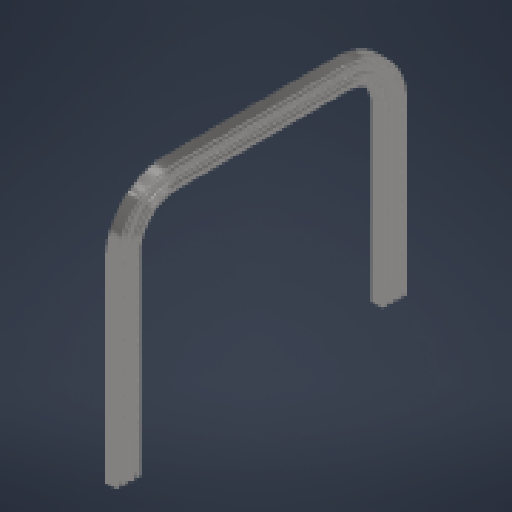
# Autodesk Inventor part: SACMI DPA C-RAIL
Saved by Autodesk Inventor 2025 (Build 290162000, 162)
## iProperties
Created: 2024-05-16
Part Number: SACMI DPA C-RAIL
Material: Generic
Document SubType Name: Modeling
Designer: zulet
Density: 1 g/cm^3
Appearance: Steel - Polished
Author: zulet
Autodesk Inventor part; units mm, degrees
ref_plane "YZ Plane" through (0, 0, 0) normal (1, 0, 0) x (0, 1, 0)
sketch "Sketch1" plane through (0, 0, 0) normal (0, 1, 0) x (-1, 0, 0)
  line L0 (0, 0) -> (-50, 0)
  line L1 (-50, 0) -> (-50, -100)
  line L2 (-50, -100) -> (0, -100)
  line L3 (0, -100) -> (0, 0)
  line L4 (-50, -90) -> (-10, -90)
  line L5 (-10, -90) -> (-10, -10)
  line L6 (-10, -10) -> (-50, -10)
  line L7 (-50, -10) -> (-50, -90) construction
  line L8 (-10, -70) -> (-50, -70)
  line L9 (-50, -70) -> (-50, -30)
  line L10 (-50, -30) -> (-10, -30)
  line L11 (-10, -30) -> (-10, -70)
  circle A0 centre (-50, -50) radius 7.5 construction
  circle A1 centre (0, -50) radius 7.5 construction
  line L12 (-49.5, -70) -> (-46.5, -70)
  line L13 (-46.5, -70) -> (-46.5, -82)
  line L14 (-46.5, -82) -> (-49.5, -82)
  line L15 (-49.5, -82) -> (-49.5, -70)
  line L16 (-50, -50) -> (0, -50) construction
  line L17 (-49.5, -10) -> (-46.5, -10)
  line L18 (-46.5, -10) -> (-46.5, -22)
  line L19 (-46.5, -22) -> (-49.5, -22)
  line L20 (-49.5, -22) -> (-49.5, -10)
  line L21 (-50, -42.5) -> (-47.5, -42.5)
  line L22 (-42.5, -47.5) -> (-42.5, -52.5)
  line L23 (-47.5, -57.5) -> (-50, -57.5)
  line L24 (-50, -57.5) -> (-50, -42.5)
  arc A2 (-47.5, -57.5) -> (-42.5, -52.5) centre (-47.5, -52.5) ccw
  arc A3 (-42.5, -47.5) -> (-47.5, -42.5) centre (-47.5, -47.5) ccw
  line L25 (-25, -100) -> (-25, 0) construction
  line L26 (0, -42.5) -> (-2.5, -42.5)
  line L27 (-7.5, -47.5) -> (-7.5, -52.5)
  line L28 (-2.5, -57.5) -> (0, -57.5)
  arc A4 (-7.5, -52.5) -> (-2.5, -57.5) centre (-2.5, -52.5) ccw
  arc A5 (-2.5, -42.5) -> (-7.5, -47.5) centre (-2.5, -47.5) ccw
  point P0 (-10, -30)
  point P1 (-50, -42.5)
  point P2 (0, -42.5)
  point P3 (-46.5, -70)
  point P4 (0, -42.5)
  point P5 (-50, -42.5)
  dimension "d2" = 15
  dimension "d0" = 50
  dimension "d1" = 100
  dimension "d3" = 40
  dimension "d4" = 10
  dimension "d5" = 10
  dimension "d6" = 10
  dimension "d7" = 15
  dimension "d66" = 3
  dimension "d67" = 12
  dimension "d68" = 0.5
  dimension "d76" = 3
  dimension "d77" = 12
  dimension "d78" = 0.5
  dimension "d82" = 5
  constraints: 58 end point, 12 parallel, 8 point on circle, 8 symmetric about line, 7 horizontal, 7 perpendicular, 6 point on line, 5 centre point, 5 midpoint, 4 tangent, 1 equal radius, 1 vertical, 5 other
  measures "d0" distance of L2.end L1.end
  measures "d1" distance of L1.end L0.end
  measures "d3" distance between parallel lines of L10 L8
  measures "d4" distance between parallel lines of L4 L2
  measures "d5" distance between parallel lines of L0 L6
  measures "d6" distance between parallel lines of L5 L3
  measures "d7" diameter of A1
  measures "d66" distance of L13.end L14.end
  measures "d67" distance of L12.end L13.end
  measures "d68" distance between parallel lines of L1 L15
  measures "d76" distance of L18.end L19.end
  measures "d77" distance of L17.end L18.end
  measures "d78" distance between parallel lines of L7 L20
  measures "d82" radius of A2
sketch "Sketch2" plane through (0, 0, 0) normal (1, 0, 0) x (0, 1, 0)
  line L0 (0, -100) -> (0, 0) projected
  line L1 (0, -50) -> (600, -50)
  line L2 (800, 150) -> (800, 850)
  line L3 (600, 1050) -> (-200, 1050)
  arc A0 (600, -50) -> (800, 150) centre (600, 150) ccw
  arc A1 (800, 850) -> (600, 1050) centre (600, 850) ccw
  point P0 (800, -50)
  dimension "d8" = 1100
  dimension "d9" = 1000
  dimension "d10" = 800
  dimension "d11" = 200
  constraints: 6 end point, 4 point on circle, 4 tangent, 2 centre point, 2 perpendicular, 2 point on line, 1 equal radius, 1 horizontal, 1 midpoint
  measures "d8" distance between parallel lines of L3 L1
  measures "d9" distance from line of L3.end L2
  measures "d10" distance of L1.start point (800, -50)
  measures "d11" radius of A0
sweep "Sweep1" add profiles "Sketch1" path "Sketch2" path curves L1 A0 L2 A1 L3 contours L3 L26 A5 L27 A4 L28 L2 L1 L4 L5 L6 L0 | L10 L5 L8 L1 L23 A2 L22 A3 L21 | L6 L18 L19 L20 | L13 L14 L15 L8
sketch "Sketch3" plane through (50, 0, -70) normal (1, 0, 0) x (0, 0, -1)
  line L0 (0, 0) -> (0, 600) projected
  line L1 (0, 0) -> (20, 0) projected
  line L2 (20, 0) -> (20, 600) construction
  line L3 (0, 600) -> (20, 600) construction
  arc A0 (0, 600) -> (-220, 820) centre (-220, 600) ccw construction
  line L4 (-220, 850) -> (-920, 850) construction
  line L5 (-570, 850) -> (-570, 760) construction
  line L6 (-220, 760) -> (-920, 760) construction
  line L7 (-220, 820) -> (-920, 820) construction
  line L8 (-220, 820) -> (-570, 820) construction
  line L9 (-27.5, 0) -> (-12.5, 0) construction
  line L10 (-20, 0) -> (-20, 600) construction
  line L11 (-27.5, 600) -> (-12.5, 600) construction
  line L12 (-220, 792.5) -> (-220, 807.5) construction
  line L13 (-220, 800) -> (-570, 800) construction
  line L14 (-70, 0) -> (30, 0) construction
  line L15 (-60, 0) -> (-60, 600) construction
  line L16 (0, 0) -> (-60, 0) construction
  line L17 (-1140, 0) -> (-1140, 600)
  line L18 (-1140, 0) -> (-1160, 0)
  line L19 (-1160, 0) -> (-1160, 600) construction
  line L20 (-1140, 600) -> (-1160, 600) construction
  arc A1 (-920, 820) -> (-1140, 600) centre (-920, 600) ccw construction
  line L21 (-920, 850) -> (-220, 850) construction
  line L22 (-920, 760) -> (-220, 760) construction
  line L23 (-920, 820) -> (-220, 820) construction
  line L24 (-920, 820) -> (-570, 820) construction
  line L25 (-1112.5, 0) -> (-1127.5, 0) construction
  line L26 (-1120, 0) -> (-1120, 600) construction
  line L27 (-1112.5, 600) -> (-1127.5, 600) construction
  line L28 (-920, 792.5) -> (-920, 807.5) construction
  line L29 (-920, 800) -> (-570, 800) construction
  line L30 (-1127.5, 0) -> (-1140, 0) construction
  line L31 (-1080, 0) -> (-1080, 600) construction
  line L32 (-1140, 0) -> (-1080, 0) construction
  line L33 (-17.5, 600) -> (-12.5, 600) projected
  line L34 (-27.5, 600) -> (-22.5, 600) projected
  line L35 (-17.5, 0) -> (-12.5, 0) projected
  line L36 (-22.5, 0) -> (-17.5, 0) projected
  line L37 (-27.5, 0) -> (-22.5, 0) projected
  line L38 (-220, 802.5) -> (-220, 807.5) projected
  line L39 (-220, 792.5) -> (-220, 797.5) projected
  line L40 (-1160, 0) -> (-1160, 600) construction
  line L41 (-220, 850) -> (-220, 760) construction
  line L42 (-1092, 600) -> (-1092, -200) projected
  point P0 (7, 25)
  point P1 (7, 600)
  point P2 (6.0317, 620.9449)
  point P3 (3.1349, 641.7111)
  point P4 (-1.6656, 662.1215)
  point P5 (-8.3288, 682.0019)
  point P6 (-16.7979, 701.1826)
  point P7 (-27.0007, 719.5001)
  point P8 (-38.8501, 736.7981)
  point P9 (-52.245, 752.9289)
  point P10 (-67.0711, 767.755)
  point P11 (-83.2019, 781.1499)
  point P12 (-100.4999, 792.9993)
  point P13 (-118.8174, 803.2021)
  point P14 (-137.9981, 811.6712)
  point P15 (-157.8785, 818.3344)
  point P16 (-178.2889, 823.1349)
  point P17 (-199.0551, 826.0317)
  point P18 (-220, 827)
  point P19 (7, 50)
  point P20 (7, 75)
  point P21 (7, 100)
  point P22 (7, 125)
  point P23 (7, 150)
  point P24 (7, 175)
  point P25 (7, 200)
  point P26 (7, 225)
  point P27 (7, 250)
  point P28 (7, 275)
  point P29 (-53, 25)
  point P30 (-53, 50)
  point P31 (-53, 75)
  point P32 (-53, 100)
  point P33 (-53, 125)
  point P34 (-53, 150)
  point P35 (-53, 175)
  point P36 (-53, 200)
  point P37 (-53, 225)
  point P38 (-53, 250)
  point P39 (-53, 275)
  point P40 (-53, 600)
  point P41 (-54.4287, 621.7979)
  point P42 (-58.6904, 643.2228)
  point P43 (-65.7121, 663.9081)
  point P44 (-75.3738, 683.5)
  point P45 (-87.51, 701.6632)
  point P46 (-101.9132, 718.0868)
  point P47 (-118.3368, 732.49)
  point P48 (-136.5, 744.6262)
  point P49 (-156.0919, 754.2879)
  point P50 (-176.7772, 761.3096)
  point P51 (-198.2021, 765.5713)
  point P52 (-220, 767)
  point P53 (-1070, 0)
  point P54 (-1147, 25)
  point P55 (-1147, 600)
  point P56 (-1146.0317, 620.9449)
  point P57 (-1143.1349, 641.7111)
  point P58 (-1138.3344, 662.1215)
  point P59 (-1131.6712, 682.0019)
  point P60 (-1123.2021, 701.1826)
  point P61 (-1112.9993, 719.5001)
  point P62 (-1101.1499, 736.7981)
  point P63 (-1087.755, 752.9289)
  point P64 (-1072.9289, 767.755)
  point P65 (-1056.7981, 781.1499)
  point P66 (-1039.5001, 792.9993)
  point P67 (-1021.1826, 803.2021)
  point P68 (-1002.0019, 811.6712)
  point P69 (-982.1215, 818.3344)
  point P70 (-961.7111, 823.1349)
  point P71 (-940.9449, 826.0317)
  point P72 (-920, 827)
  point P73 (-1147, 50)
  point P74 (-1147, 75)
  point P75 (-1147, 100)
  point P76 (-1147, 125)
  point P77 (-1147, 150)
  point P78 (-1147, 175)
  point P79 (-1147, 200)
  point P80 (-1147, 225)
  point P81 (-1147, 250)
  point P82 (-1147, 275)
  point P83 (-1087, 25)
  point P84 (-1087, 50)
  point P85 (-1087, 75)
  point P86 (-1087, 100)
  point P87 (-1087, 125)
  point P88 (-1087, 150)
  point P89 (-1087, 175)
  point P90 (-1087, 200)
  point P91 (-1087, 225)
  point P92 (-1087, 250)
  point P93 (-1087, 275)
  point P94 (-1087, 600)
  point P95 (-1085.5713, 621.7979)
  point P96 (-1081.3096, 643.2228)
  point P97 (-1074.2879, 663.9081)
  point P98 (-1064.6262, 683.5)
  point P99 (-1052.49, 701.6632)
  point P100 (-1038.0868, 718.0868)
  point P101 (-1021.6632, 732.49)
  point P102 (-1003.5, 744.6262)
  point P103 (-983.9081, 754.2879)
  point P104 (-963.2228, 761.3096)
  point P105 (-941.7979, 765.5713)
  point P106 (-920, 767)
  point P107 (7, 300)
  point P108 (-53, 300)
  point P109 (7, 325)
  point P110 (-53, 325)
  point P111 (7, 350)
  point P112 (-53, 350)
  point P113 (7, 375)
  point P114 (-53, 375)
  point P115 (7, 400)
  point P116 (-53, 400)
  point P117 (7, 425)
  point P118 (-53, 425)
  point P119 (7, 450)
  point P120 (-53, 450)
  point P121 (7, 475)
  point P122 (-53, 475)
  point P123 (7, 500)
  point P124 (-53, 500)
  point P125 (7, 525)
  point P126 (-53, 525)
  point P127 (7, 550)
  point P128 (-53, 550)
  point P129 (7, 575)
  point P130 (-53, 575)
  point P131 (-1147, 275)
  point P132 (-1087, 275)
  point P133 (-1147, 300)
  point P134 (-1087, 300)
  point P135 (-1147, 325)
  point P136 (-1087, 325)
  point P137 (-1147, 350)
  point P138 (-1087, 350)
  point P139 (-1147, 375)
  point P140 (-1087, 375)
  point P141 (-1147, 400)
  point P142 (-1087, 400)
  point P143 (-1147, 425)
  point P144 (-1087, 425)
  point P145 (-1147, 450)
  point P146 (-1087, 450)
  point P147 (-1147, 475)
  point P148 (-1087, 475)
  point P149 (-1147, 500)
  point P150 (-1087, 500)
  point P151 (-1147, 525)
  point P152 (-1087, 525)
  point P153 (-1147, 550)
  point P154 (-1087, 550)
  point P155 (-1147, 575)
  point P156 (-1087, 575)
  point P157 (-1147, 600)
  point P158 (-1087, 600)
  point P159 (-245, 827)
  point P160 (-270, 827)
  point P161 (-295, 827)
  point P162 (-320, 827)
  point P163 (-345, 827)
  point P164 (-370, 827)
  point P165 (-395, 827)
  point P166 (-420, 827)
  point P167 (-445, 827)
  point P168 (-470, 827)
  point P169 (-245, 767)
  point P170 (-270, 767)
  point P171 (-295, 767)
  point P172 (-320, 767)
  point P173 (-345, 767)
  point P174 (-370, 767)
  point P175 (-395, 767)
  point P176 (-420, 767)
  point P177 (-445, 767)
  point P178 (-470, 767)
  point P179 (-895, 827)
  point P180 (-870, 827)
  point P181 (-845, 827)
  point P182 (-820, 827)
  point P183 (-795, 827)
  point P184 (-770, 827)
  point P185 (-745, 827)
  point P186 (-720, 827)
  point P187 (-695, 827)
  point P188 (-895, 767)
  point P189 (-870, 767)
  point P190 (-845, 767)
  point P191 (-820, 767)
  point P192 (-795, 767)
  point P193 (-770, 767)
  point P194 (-745, 767)
  point P195 (-720, 767)
  point P196 (-695, 767)
  point P197 (-495, 827)
  point P198 (-495, 767)
  point P199 (-520, 827)
  dimension "d14" = 7
  dimension "d15" = 25
  dimension "d23" = 600
  dimension "d24" = 7
  dimension "d27" = 90
  dimension "d37" = 350
  dimension "d38" = 60
  dimension "d41" = 25
  dimension "d44" = 60
  dimension "d57" = 60
  dimension "d64" = 90
  dimension "d85" = 25
  dimension "d88" = 60
  dimension "d91" = 25
  dimension "d92" = 7
  dimension "d94" = 7
  dimension "d97" = 25
  dimension "d100" = 60
  constraints: 128 symmetric about line, 54 end point, 6 midpoint, 5 horizontal, 5 vertical, 4 point on line, 2 perpendicular, 2 point on circle, 1 centre point, 120 other
  measures "d14" distance from line of L0 point (7, 25)
  measures "d15" distance from line of L1 point (7, 25)
  measures "d23" distance of L0.start L0.end
  measures "d24" distance from line of L0 point (7, 600)
  measures "d37" distance of L7.start L8.end
  measures "d38" distance of L0.start L15.start
  measures "d41" distance of point (7, 25) point (7, 50)
  measures "d44" distance of point (7, 25) point (-53, 25)
  measures "d57" distance of point (7, 600) point (-53, 600)
  measures "d85" distance of point (-245, 827) point (-270, 827)
  measures "d88" distance of point (-245, 827) point (-245, 767)
  measures "d91" distance from line of point (-245, 827) L41
  measures "d92" distance from line of L23 point (-245, 827)
  measures "d94" distance from line of L31 point (-1087, 0)
  measures "d97" distance of point (-1087, 0) point (-1087, -25)
  measures "d100" distance of point (-1087, 0) point (-1147, 0)
hole "Hole1" at (50, 25, -77) direction (-1, 0, 0) diameter 4 end through all
fillet "Fillet1" radius 2 20 edges at (0, 300, -100) (0, 200, 1100) (0, 776.7767, 1026.7767) (0, 850, 500) (0, 776.7767, -26.7767) (50, 300, -100) (50, 776.7767, -26.7767) (50, 850, 500) (50, 776.7767, 1026.7767) (50, 200, 1100) (50, 300, 0) (50, 200, 1000) (50, 706.066, 956.066) (50, 750, 500) (50, 706.066, 43.934) (0, 300, 0) (0, 706.066, 43.934) (0, 750, 500) (0, 706.066, 956.066) (0, 200, 1000)
fillet "Fillet2" radius 2 20 edges at (10, 300, -70) (10, 200, 1070) (10, 755.5635, 1005.5635) (10, 820, 500) (10, 755.5635, -5.5635) (10, 300, -10) (10, 200, 1010) (10, 713.1371, 963.1371) (10, 760, 500) (10, 713.1371, 36.8629) (10, 300, -30) (10, 727.2792, 22.7208) (10, 780, 500) (10, 727.2792, 977.2792) (10, 200, 1030) (10, 300, -90) (10, 769.7056, -19.7056) (10, 840, 500) (10, 769.7056, 1019.7056) (10, 200, 1090)
pattern_sketch "Sketch Driven Pattern1" of "Hole1" from (50, 25, -77) copies at (50, 600, -77) at (50, 620.9449, -76.0317) at (50, 641.7111, -73.1349) at (50, 662.1215, -68.3344) at (50, 682.0019, -61.6712) at (50, 701.1826, -53.2021) at (50, 719.5001, -42.9993) at (50, 736.7981, -31.1499) at (50, 752.9289, -17.755) at (50, 767.755, -2.9289) at (50, 781.1499, 13.2019) at (50, 792.9993, 30.4999) at (50, 803.2021, 48.8174) at (50, 811.6712, 67.9981) at (50, 818.3344, 87.8785) at (50, 823.1349, 108.2889) at (50, 826.0317, 129.0551) at (50, 827, 150) at (50, 50, -77) at (50, 75, -77) at (50, 100, -77) at (50, 125, -77) at (50, 150, -77) at (50, 175, -77) at (50, 200, -77) at (50, 225, -77) at (50, 250, -77) at (50, 275, -77) at (50, 25, -17) at (50, 50, -17) at (50, 75, -17) at (50, 100, -17) at (50, 125, -17) at (50, 150, -17) at (50, 175, -17) at (50, 200, -17) at (50, 225, -17) at (50, 250, -17) at (50, 275, -17) at (50, 600, -17) at (50, 621.7979, -15.5713) at (50, 643.2228, -11.3096) at (50, 663.9081, -4.2879) at (50, 683.5, 5.3738) at (50, 701.6632, 17.51) at (50, 718.0868, 31.9132) at (50, 732.49, 48.3368) at (50, 744.6262, 66.5) at (50, 754.2879, 86.0919) at (50, 761.3096, 106.7772) at (50, 765.5713, 128.2021) at (50, 767, 150) at (50, 767, 850) at (50, 765.5713, 871.7979) at (50, 761.3096, 893.2228) at (50, 754.2879, 913.9081) at (50, 744.6262, 933.5) at (50, 732.49, 951.6632) at (50, 718.0868, 968.0868) at (50, 701.6632, 982.49) at (50, 683.5, 994.6262) at (50, 663.9081, 1004.2879) at (50, 643.2228, 1011.3096) at (50, 621.7979, 1015.5713) at (50, 600, 1017) at (50, 275, 1017) at (50, 250, 1017) at (50, 225, 1017) at (50, 200, 1017) at (50, 175, 1017) at (50, 150, 1017) at (50, 125, 1017) at (50, 100, 1017) at (50, 75, 1017) at (50, 50, 1017) at (50, 25, 1017) at (50, 275, 1077) at (50, 250, 1077) at (50, 225, 1077) at (50, 200, 1077) at (50, 175, 1077) at (50, 150, 1077) at (50, 125, 1077) at (50, 100, 1077) at (50, 75, 1077) at (50, 50, 1077) at (50, 827, 850) at (50, 826.0317, 870.9449) at (50, 823.1349, 891.7111) at (50, 818.3344, 912.1215) at (50, 811.6712, 932.0019) at (50, 803.2021, 951.1826) at (50, 792.9993, 969.5001) at (50, 781.1499, 986.7981) at (50, 767.755, 1002.9289) at (50, 752.9289, 1017.755) at (50, 736.7981, 1031.1499) at (50, 719.5001, 1042.9993) at (50, 701.1826, 1053.2021) at (50, 682.0019, 1061.6712) at (50, 662.1215, 1068.3344) at (50, 641.7111, 1073.1349) at (50, 620.9449, 1076.0317) at (50, 600, 1077) at (50, 25, 1077) at (50, 300, -77) at (50, 300, -17) at (50, 325, -77) at (50, 325, -17) at (50, 350, -77) at (50, 350, -17) at (50, 375, -77) at (50, 375, -17) at (50, 400, -77) at (50, 400, -17) at (50, 425, -77) at (50, 425, -17) at (50, 450, -77) at (50, 450, -17) at (50, 475, -77) at (50, 475, -17) at (50, 500, -77) at (50, 500, -17) at (50, 525, -77) at (50, 525, -17) at (50, 550, -77) at (50, 550, -17) at (50, 575, -77) at (50, 575, -17) at (50, 575, 1017) at (50, 575, 1077) at (50, 550, 1017) at (50, 550, 1077) at (50, 525, 1017) at (50, 525, 1077) at (50, 500, 1017) at (50, 500, 1077) at (50, 475, 1017) at (50, 475, 1077) at (50, 450, 1017) at (50, 450, 1077) at (50, 425, 1017) at (50, 425, 1077) at (50, 400, 1017) at (50, 400, 1077) at (50, 375, 1017) at (50, 375, 1077) at (50, 350, 1017) at (50, 350, 1077) at (50, 300, 1017) at (50, 300, 1077) at (50, 325, 1017) at (50, 325, 1077) at (50, 827, 175) at (50, 827, 200) at (50, 827, 225) at (50, 827, 250) at (50, 827, 275) at (50, 827, 300) at (50, 827, 325) at (50, 827, 350) at (50, 827, 375) at (50, 827, 400) at (50, 767, 175) at (50, 767, 200) at (50, 767, 225) at (50, 767, 250) at (50, 767, 275) at (50, 767, 300) at (50, 767, 325) at (50, 767, 350) at (50, 767, 375) at (50, 767, 400) at (50, 767, 625) at (50, 767, 650) at (50, 767, 675) at (50, 767, 700) at (50, 767, 725) at (50, 767, 750) at (50, 767, 775) at (50, 767, 800) at (50, 767, 825) at (50, 827, 625) at (50, 827, 650) at (50, 827, 675) at (50, 827, 700) at (50, 827, 725) at (50, 827, 750) at (50, 827, 775) at (50, 827, 800) at (50, 827, 825) at (50, 827, 425) at (50, 767, 425) at (50, 827, 450) at (50, 767, 450) at (50, 827, 475) at (50, 767, 475) at (50, 827, 500) at (50, 767, 500) at (50, 767, 525) at (50, 827, 525) at (50, 767, 550) at (50, 827, 550) at (50, 767, 575) at (50, 827, 575) at (50, 767, 600) at (50, 827, 600) at (50, 0, 1017) at (50, -25, 1017) at (50, -50, 1017) at (50, -75, 1017) at (50, 0, 1077) at (50, -25, 1077) at (50, -50, 1077) at (50, -75, 1077) at (50, -100, 1017) at (50, -100, 1077) at (50, -125, 1017) at (50, -125, 1077) at (50, -150, 1017) at (50, -150, 1077) at (50, -175, 1017) at (50, -175, 1077)
ref_plane "Work Plane1" through (25, 0, -70) normal (1, 0, 0) x (0, 0, -1)
ref_plane "Work Plane2" through (48, 0, -50) normal (0, 0, -1) x (-1, 0, 0)
equation "\"d5\" = d4"
equation "\"d6\" = d4"
equation "\"d7\" = d2"
equation "\"d15\" = spacing"
equation "\"d24\" = d14"
equation "\"d41\" = spacing"
equation "\"d44\" = d38"
equation "\"d57\" = d38"
equation "\"d85\" = spacing"
equation "\"d88\" = d38"
equation "\"d91\" = spacing"
equation "\"d92\" = d14"
equation "\"d94\" = d14"
equation "\"d97\" = spacing"
equation "\"d100\" = d38"
equation "\"spacing\" = 25"
body "Solid1"
